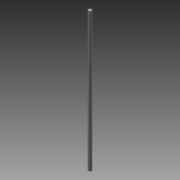
# Autodesk Inventor part: rod
Saved by Autodesk Inventor 2016 (Build 200138000, 138)
## iProperties
Created: 2016-01-27
Part Number: rod
Material: Generic
Document SubType Name: Modeling
Designer: 278648
Density: 1 g/cm^3
Appearance: Default
Mass: 78.0539 g
Surface Area: 248.633 cm^2
Volume: 78.0539 cm^3
Author: 278648
Autodesk Inventor part; units mm, degrees
ref_plane "YZ Plane" through (0, 0, 0) normal (1, 0, 0) x (0, 1, 0)
ref_plane "XZ Plane" through (0, 0, 0) normal (0, 1, 0) x (-1, 0, 0)
ref_plane "XY Plane" through (0, 0, 0) normal (0, 0, 1) x (1, 0, 0)
sketch "Sketch1" plane through (0, 0, 0) normal (0, 1, 0) x (-1, 0, 0)
  line L0 (-3.6086, 6.3829) -> (3.7235, 6.3166)
  line L1 (3.7235, 6.3166) -> (7.332, -0.0663)
  line L2 (7.332, -0.0663) -> (3.6086, -6.3829)
  line L3 (3.6086, -6.3829) -> (-3.7235, -6.3166)
  line L4 (-3.7235, -6.3166) -> (-7.332, 0.0663)
  line L5 (-7.332, 0.0663) -> (-3.6086, 6.3829)
  point P0 (0, 0)
  point P1 (0, 0)
  dimension "d0" = 12.7
  constraints: 12 end point, 1 coincident, 13 other
  measures "d0" distance between parallel lines of L3 L0
extrude "Extrusion1" add sketch "Sketch1" along normal blind 558.8
body "Solid1"
